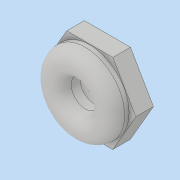
# Autodesk Inventor part: sealNut
Saved by Autodesk Inventor 2017 (Build 210142000, 142)
## iProperties
Created: 2016-10-25
Part Number: sealNut
Material: Generic
Document SubType Name: Modeling
Designer: techn
Density: 1 g/cm^3
Appearance: Default
Author: techn
Autodesk Inventor part; units mm, degrees
ref_plane "YZ Plane" through (0, 0, 0) normal (1, 0, 0) x (0, 1, 0)
ref_plane "XZ Plane" through (0, 0, 0) normal (0, 1, 0) x (-1, 0, 0)
ref_plane "XY Plane" through (0, 0, 0) normal (0, 0, 1) x (1, 0, 0)
sketch "Sketch2" plane through (0, 0, 0) normal (0, 0, 1) x (1, 0, 0)
  line L0 (-5.1962, 0) -> (-2.5981, 4.5)
  line L1 (-2.5981, 4.5) -> (2.5981, 4.5)
  line L2 (2.5981, 4.5) -> (5.1962, 0)
  line L3 (5.1962, 0) -> (2.5981, -4.5)
  line L4 (2.5981, -4.5) -> (-2.5981, -4.5)
  line L5 (-2.5981, -4.5) -> (-5.1962, 0)
  point P0 (0, 0)
  point P1 (0, 0)
  dimension "d0" = 9
  constraints: 12 end point, 1 coincident, 13 other
  measures "d0" distance between parallel lines of L4 L1
extrude "Extrusion1" add sketch "Sketch2" along normal blind 2
sketch "Sketch3" plane through (0, 0, 0) normal (0, 1, 0) x (-1, 0, 0)
  line L0 (5.1962, 0) -> (5.1962, 2) projected
  line L1 (2.5981, 2) -> (-2.5981, 2) projected
  line L2 (0, 2) -> (1.585, 2)
  line L3 (2.5981, 2) -> (5.1962, 2) projected
  line L4 (5.1962, 2) -> (4.4462, 2)
  line L5 (1.585, 2) -> (1.585, 2.5)
  line L6 (4.4462, 2) -> (4.4462, 2.5)
  arc A0 (4.4462, 2.5) -> (1.585, 2.5) centre (3.0156, 2.5) ccw
  line L7 (0, 2) -> (0, 5.5151)
  point P0 (0, 0)
  dimension "d3" = 1.585
  dimension "d4" = 0.75
  dimension "d5" = 0.5
  dimension "d6" = 0.5
  constraints: 10 end point, 3 vertical, 2 point on circle, 2 point on line, 1 centre point, 1 midpoint, 1 tangent
  measures "d3" distance of L2.start L2.end
  measures "d4" distance of L0.end L4.end
  measures "d5" distance of L2.end L5.end
  measures "d6" distance of L4.end L6.end
revolve "Revolution1" add sketch "Sketch3" angle 360 about axis through (0, 0, 2) along (0, 0, 1)
sketch "Sketch4" plane through (0, 0, 2) normal (0, 0, 1) x (1, 0, 0)
  circle A0 centre (0, 0) radius 1.585 projected
  point P0 (0, 0)
extrude "Extrusion2" cut sketch "Sketch4" against normal through all
sketch "Sketch5" plane through (0, 0, 0) normal (0, 0, -1) x (-1, 0, 0)
  circle A0 centre (0, 0) radius 3
  dimension "d10" = 6
  constraints: 1 centre point, 1 coincident
  measures "d10" diameter of A0
extrude "Extrusion3" cut sketch "Sketch5" against normal blind 1.5
body "Solid1"
